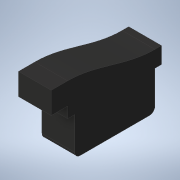
# Autodesk Inventor part: canopy
Saved by Autodesk Inventor 2020 (Build 240168000, 168)
## iProperties
Part Number: canopy
Material: GEDA Polyamid schwarz
Document SubType Name: Modeling
Designer: Admin
Mass: 1220.8 g
Surface Area: 691.534 cm^2
Volume: 1070.88 cm^3
Density: 1.14 g/cm^3
Appearance: GEDA Plastik schwarz A
Gewicht: 1,221 kg
G_L: 0
G_H: 0
G_B: 0
InventorVersion: 2019.4
VAULT_Status: in Bearbeitung
Revision: -
Max. Breite: 0
Max. Höhe: 0
Max. Länge: 0
Max. Abmessungen: 0 x 0 x 0
Author: Admin
Autodesk Inventor part; units mm, degrees
note: some values were not read from the file. Left out: dimensions or parameters whose unit could not be read.
ref_plane "YZ Plane" through (0, 0, 0) normal (1, 0, 0) x (0, 1, 0)
ref_plane "XZ Plane" through (0, 0, 0) normal (0, 1, 0) x (-1, 0, 0)
ref_plane "XY Plane" through (0, 0, 0) normal (0, 0, 1) x (1, 0, 0)
sketch "Skizze1" plane through (0, 0, 0) normal (0, 0, 1) x (1, 0, 0)
  line L0 (-30, -80) -> (30, -80)
  line L1 (30, -80) -> (30, 80)
  line L2 (30, 80) -> (-30, 80)
  line L3 (-30, 80) -> (-30, -80)
  line L4 (-30, -80) -> (30, 80) construction
  line L5 (30, -80) -> (-30, 80) construction
  point P0 (0, 0)
  dimension "d0" = 60
  dimension "d1" = 160
  constraints: 12 end point, 2 midpoint, 2 parallel, 1 horizontal, 1 perpendicular
  measures "d0" distance of L2.end L1.end
  measures "d1" distance of L1.end L0.end
extrude "Extrusion1" add sketch "Skizze1" along normal blind 100
sketch "Skizze2" plane through (30, -80, 0) normal (1, 0, 0) x (0, 0, -1)
  line L0 (-100, 160) -> (-100, 0) projected
  line L1 (0, 0) -> (-100, 0) projected
  line L2 (-100, 160) -> (-100, 0)
  line L3 (-100, 0) -> (-130, 0)
  spline S0 degree 4 poles (-130, 0) (-130, 41.0456) (-115, 80) (-100, 118.9544) (-100, 160) knots 0 0 0 0 0 1 1 1 1 1
  point P0 (0, 80)
  point P1 (-115, 80)
  point P2 (-100, 80)
  point P3 (-115, 0)
  dimension "d4" = 30
  constraints: 4 end point, 2 midpoint, 2 vertical, 1 horizontal, 1 horizontal alignment, 1 perpendicular, 1 vertical alignment, 3 other
  measures "d4" distance of L0.end L3.end
extrude "Extrusion2" add sketch "Skizze2" against normal up to surface (60 mm away)
sketch "Skizze5" plane through (30, -80, 0) normal (1, 0, 0) x (0, 0, -1)
  line L0 (0, 0) -> (-70, 0)
  line L1 (-70, 0) -> (-70, 13)
  line L2 (-70, 13) -> (0, 13)
  line L3 (0, 13) -> (0, 0)
  point P0 (0, 80)
  dimension "d15" = 70
  dimension "d16" = 13
  constraints: 8 end point, 2 parallel, 1 horizontal, 1 perpendicular
  measures "d15" distance of L1.end L2.end
  measures "d16" distance of L0.end L1.end
extrude "Extrusion5" cut sketch "Skizze5" against normal through all
sketch "Skizze6" plane through (30, 80, 100) normal (1, 0, 0) x (0, 0, -1)
  line L0 (30, -160) -> (-30, -160) projected
  line L1 (10, -160) -> (10, -190)
  line L2 (10, -190) -> (-30, -190)
  line L3 (-30, -190) -> (-30, -160)
  line L4 (30, -160) -> (30, -147) projected
  line L5 (100, 0) -> (0, 0) projected
  line L6 (0, 0) -> (30, 0)
  line L7 (30, 0) -> (30, 12)
  line L8 (30, 12) -> (0, 12)
  line L9 (0, 12) -> (0, 0)
  point P0 (100, -80)
  point P1 (30, 0)
  dimension "d19" = 20
  dimension "d20" = 40
  dimension "d21" = 30
  dimension "d24" = 30
  dimension "d25" = 12
  constraints: 14 end point, 3 parallel, 2 perpendicular, 1 horizontal, 1 point on line
  measures "d19" distance from line of L4 L1.start
  measures "d20" distance of L1.end L2.end
  measures "d21" distance of L2.end L0.end
  measures "d24" distance of L8.end L7.end
  measures "d25" distance of L7.end L6.end
extrude "Extrusion6" add sketch "Skizze6" against normal up to surface (60 mm away)
fillet "Rundung1" radius 10 2 edges at (0, -67, 0) (0, 80, 0)
equation "\"G_L\" = 0"
equation "\"G_H\" = 0"
equation "\"G_B\" = 0"
